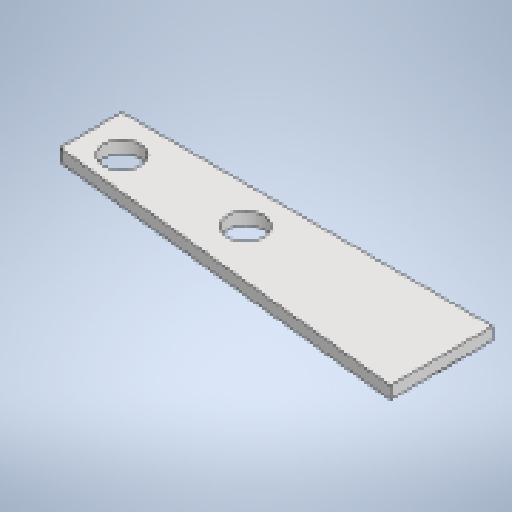
# Autodesk Inventor part: TRM 030 star conrtforce plate
Saved by Autodesk Inventor 2025.1 (Build 291241020, 241B)
## iProperties
Created: 2024-08-07
Part Number: TRM 030 star conrtforce plate
Material: AISI 304
Document SubType Name: Sheet Metal
Designer: admin
Stock Number: ТРМ 015 левый борт основное
Density: 8.02768 g/cm^3
Flat Pattern Width: 6 cm
Flat Pattern Length: 1.65934 cm
Flat Pattern Area: 9.95604 cm^2
Sheet Metal Rule: AISI304 2mm Die16
Sheet Metal Width: 60.000 mm
Sheet Metal Length: 16.593 mm
Sheet Metal Area: 995.604 mm^2
Appearance: Default
Mass: 57.5336 g
Surface Area: 80.5249 cm^2
Volume: 7.1669 cm^3
Author: pokla
Autodesk Inventor part; units mm, degrees
ref_plane "YZ Plane" through (0, 0, 0) normal (1, 0, 0) x (0, 1, 0)
ref_plane "XZ Plane" through (0, 0, 0) normal (0, 1, 0) x (-1, 0, 0)
ref_plane "XY Plane" through (0, 0, 0) normal (0, 0, 1) x (1, 0, 0)
sketch "Sketch1" plane through (0, 0, 0) normal (0, 0, 1) x (1, 0, 0)
  line L0 (60, 0) -> (60, -16.5934)
  line L1 (60, 0) -> (0, 0)
  line L2 (0, 0) -> (0, -10)
  line L3 (0, -10) -> (60, -16.5934)
  dimension "d43" = 10
  dimension "d44" = 60
  dimension "d51" = 6.271
  measures "d43" distance of L1.end L2.end
  measures "d44" distance of L0.start L1.end
  measures "d51" angle of L1 L3
extrude "Plate1" add sketch "Sketch1" along normal blind 2
sketch "Sketch6" plane through (0, 0, 0) normal (0, 0, 1) x (1, 0, 0)
  line L0 (0, -10) -> (60, -16.5934) projected
  line L1 (0, 0) -> (0, -10) projected
  line L2 (60, 0) -> (0, 0) projected
  line L3 (60, -16.5934) -> (60, 0) projected
  circle A0 centre (6, -6) radius 3
  circle A1 centre (26, -6) radius 3
  dimension "d45" = 6
  dimension "d46" = 6
  dimension "d47" = 6
  dimension "d48" = 20
  constraints: 2 centre point, 1 equal radius, 1 horizontal alignment
  measures "d45" distance from line of A0.centre L2
  measures "d46" distance from line of A0.centre L1
  measures "d47" diameter of A0
  measures "d48" distance of A1.centre A0.centre
sketch "Sketch2" plane through (0, 0, 0) normal (0, 0, -1) x (-1, 0, 0)
  line L0 (-179.9406, -4.4713) -> (20.0594, -4.4713) construction
  line L1 (20.0594, -4.4713) -> (20.0594, -24.4713) construction
  line L2 (20.0594, -24.4713) -> (-179.9406, -24.4713) construction
  line L3 (-179.9406, -24.4713) -> (-179.9406, -4.4713) construction
  point P0 (0, 0)
  point P1 (-251, -525)
  dimension "d6" = 200
  dimension "d9" = 20
  constraints: 2 other
  measures "d6" distance of L0.start L0.end
  measures "d9" distance of L0.end L1.end
mark "Mark1"
extrude "Extrusion1" cut sketch "Sketch6" along normal through all contours A0 | A1
equation "\"d2\" = Thickness"
equation "\"BendReliefWidth\" = Thickness"
equation "\"BendReliefDepth\" = 0.5 * Thickness"
equation "\"CornerReliefSize\" = 4 * Thickness"
equation "\"MinimumRemnant\" = 2 * Thickness"
equation "\"TransitionRadius\" = BendRadius"
equation "\"JacobiRadiusSize\" = BendRadius"
equation "\"GapSize\" = Thickness"
equation "\"Thickness\" = 2"
equation "\"BendRadius\" = 2.75"
body "Solid1"
